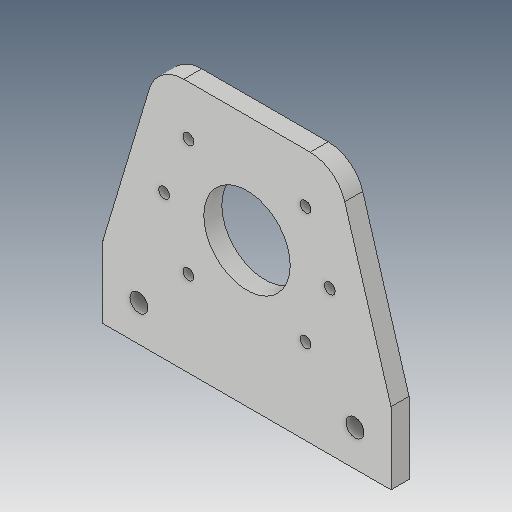
# Autodesk Inventor part: 車軸受け板
Saved by Autodesk Inventor 2020.3 (Build 243373000, 373)
## iProperties
Part Number: 車軸受け板
Material: 一般
Document SubType Name: Modeling
Designer: highs
Density: 1 g/cm^3
Appearance: 既定
Author: highs
Autodesk Inventor part; units mm, degrees
ref_plane "YZ Plane" through (0, 0, 0) normal (1, 0, 0) x (0, 1, 0)
ref_plane "XZ Plane" through (0, 0, 0) normal (0, 1, 0) x (-1, 0, 0)
ref_plane "XY Plane" through (0, 0, 0) normal (0, 0, 1) x (1, 0, 0)
sketch "スケッチ1" plane through (0, 0, 0) normal (0, 0, 1) x (1, 0, 0)
  line L0 (0, 0) -> (80, 0)
  line L1 (80, 0) -> (80, 20)
  line L2 (40, 0) -> (40, 153.3333) construction
  line L3 (0, 20) -> (0, 0)
  line L4 (0, 20) -> (15, 70)
  line L5 (65, 70) -> (80, 20)
  circle A0 centre (40, 40) radius 12
  line L6 (0, 10) -> (80, 10) construction
  circle A1 centre (10, 10) radius 2.5
  circle A2 centre (70, 10) radius 2.5
  line L7 (40, 40) -> (63.0125, 40) construction
  circle A3 centre (63.0125, 40) radius 1.5
  circle A4 centre (16.9875, 40) radius 1.5
  circle A5 centre (40, 40) radius 13.25 construction
  line L8 (15, 70) -> (65, 70)
  circle A6 centre (40, 40) radius 23.0125 construction
  line L9 (23.7277, 56.2723) -> (56.2723, 23.7277) construction
  circle A7 centre (56.2723, 23.7277) radius 1.5
  circle A8 centre (23.7277, 56.2723) radius 1.5
  circle A9 centre (56.2723, 56.2723) radius 1.5
  circle A10 centre (23.7277, 23.7277) radius 1.5
  dimension "d0" = 20
  dimension "d2" = 80
  dimension "d5" = 24
  dimension "d6" = 5
  dimension "d7" = 10
  dimension "d10" = 23.0125
  dimension "d11" = 3
  dimension "d12" = 26.5
  dimension "d13" = 40
  dimension "d14" = 30
  dimension "d16" = 50
  dimension "d18" = 45
  constraints: 20 end point, 11 centre point, 5 coincident, 4 midpoint, 4 point on line, 4 symmetric about line, 3 horizontal, 3 point on circle, 2 equal radius, 1 parallel, 1 perpendicular, 1 vertical, 5 other
  measures "d0" distance of L3.start L0.start
  measures "d2" distance of L0.start L0.end
  measures "d5" diameter of A0
  measures "d6" diameter of A1
  measures "d7" distance from line of L3 A1.centre
  measures "d10" distance of L7.start L7.end
  measures "d11" diameter of A3
  measures "d12" diameter of A5
  measures "d13" distance from line of L0 L7.start
  measures "d14" distance from line of L8 A5.centre
  measures "d16" distance of L4.end L5.start
  measures "d18" angle of L7 L9
extrude "押し出し1" add sketch "スケッチ1" along normal blind 5
fillet "フィレット1" radius 10 2 edges at (65, 70, 2.5) (15, 70, 2.5)
